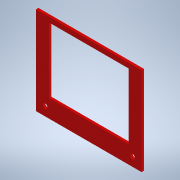
# Autodesk Inventor part: lag2
Saved by Autodesk Inventor 2022 (Build 260153000, 153)
## iProperties
Created: 2023-08-31
Part Number: lag2
Material: Generic
Document SubType Name: Modeling
Designer: THK
Density: 1 g/cm^3
Appearance: Red
Author: THK
Autodesk Inventor part; units mm, degrees
ref_plane "YZ Plane" through (0, 0, 0) normal (1, 0, 0) x (0, 1, 0)
ref_plane "XZ Plane" through (0, 0, 0) normal (0, 1, 0) x (-1, 0, 0)
ref_plane "XY Plane" through (0, 0, 0) normal (0, 0, 1) x (1, 0, 0)
sketch "Sketch1" plane through (0, 0, 0) normal (0, 0, 1) x (1, 0, 0)
  line L0 (199, 195.1016) -> (-199, 195.1016) projected
  line L1 (-199, 195.1016) -> (-199, -130.8984) projected
  line L2 (-199, -130.8984) -> (199, -130.8984) projected
  line L3 (199, -130.8984) -> (199, 195.1016) projected
  line L4 (-264.1156, 220.8859) -> (-264.1156, -220.8859) projected
  line L5 (-264.1156, -220.8859) -> (264.1156, -220.8859) projected
  line L6 (264.1156, -220.8859) -> (264.1156, 220.8859) projected
  line L7 (264.1156, 220.8859) -> (-264.1156, 220.8859) projected
  line L8 (-200, 196.1016) -> (200, 196.1016)
  line L9 (200, 196.1016) -> (200, -131.8984)
  line L10 (200, -131.8984) -> (-200, -131.8984)
  line L11 (-200, -131.8984) -> (-200, 196.1016)
  point P0 (0, 0)
  dimension "d0" = 1
  constraints: 8 end point, 3 other
  measures "d0" distance between parallel lines of L0 L8
extrude "Extrusion1" add sketch "Sketch1" along normal blind 12 contours L7 L6 L5 L4
sketch "Sketch2" plane through (0, 0, 0) normal (0, 0, -1) x (-1, 0, 0)
  point P0 (0, 0)
  point P1 (-219.1094, -175.8797)
  point P2 (219.1094, -175.8797)
hole "Hole1" at (219.1094, -175.8797, 0) at (-219.1094, -175.8797, 0) direction (0, 0, 1) diameter 23 end through all
body "Solid1"
